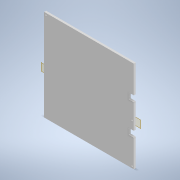
# Autodesk Inventor part: CoverPSU
Saved by Autodesk Inventor 2022 (Build 260153000, 153)
## iProperties
Created: 2022-01-15
Part Number: CoverPSU
Material: Generic
Document SubType Name: Modeling
Designer: siwat
Density: 1 g/cm^3
Appearance: Default
VLDS_Profile: Default Part
VLDS_TimeStamp: 2022-02-27
VLDS_FailCnt: 1
VLDS_AcceptCnt: 0
Author: siwat
Autodesk Inventor part; units mm, degrees
ref_plane "YZ Plane" through (0, 0, 0) normal (1, 0, 0) x (0, 1, 0)
ref_plane "XZ Plane" through (0, 0, 0) normal (0, 1, 0) x (-1, 0, 0)
ref_plane "XY Plane" through (0, 0, 0) normal (0, 0, 1) x (1, 0, 0)
ref_plane "Work Plane1" through (0, 0, 0) normal (0, 0, 1) x (1, 0, 0)
sketch "Sketch1" plane through (0, 0, 0) normal (0, 0, 1) x (1, 0, 0)
  line L0 (67.3785, -57.1866) -> (-67.4215, -57.1866)
  line L1 (-67.4215, -57.1866) -> (-67.4215, 80.2134)
  line L2 (-67.4215, 80.2134) -> (67.3785, 80.2134)
  line L3 (67.3785, 80.2134) -> (67.3785, -57.1866)
  circle A0 centre (64.6972, 5.0885) radius 1
  circle A1 centre (-64.8231, 77.3114) radius 1
  circle A2 centre (64.7712, -54.4524) radius 1
  point P0 (0, 0)
  dimension "d0" = 2
  dimension "d1" = 2
  dimension "d4" = 2
  dimension "d11" = 137.4
  dimension "d12" = 134.8
  constraints: 8 end point, 3 centre point, 2 parallel, 1 horizontal, 1 perpendicular
  measures "d0" diameter of A0
  measures "d1" diameter of A1
  measures "d4" diameter of A2
  measures "d11" distance of L2.end L0.start
  measures "d12" distance of L1.end L2.end
extrude "Extrusion1" add sketch "Sketch1" along normal blind 3
sketch "Sketch2" plane through (0, 0, 3) normal (0, 0, 1) x (1, 0, 0)
  line L0 (67.3785, -57.1866) -> (67.3785, 80.2134) projected
  line L1 (67.3785, -16.1531) -> (59.3785, -16.1531)
  line L2 (59.3785, -16.1531) -> (59.3785, -7.1531)
  line L3 (59.3785, -7.1531) -> (67.3785, -7.1531)
  line L4 (67.3785, -7.1531) -> (67.3785, -16.1531)
  line L5 (67.3785, 29.9305) -> (59.3785, 29.9305)
  line L6 (59.3785, 29.9305) -> (59.3785, 38.9305)
  line L7 (59.3785, 38.9305) -> (67.3785, 38.9305)
  line L8 (67.3785, 38.9305) -> (67.3785, 29.9305)
  point P0 (0, 0)
  dimension "d5" = 8
  dimension "d6" = 9
  dimension "d7" = 8
  dimension "d8" = 9
  constraints: 16 end point, 4 parallel, 2 horizontal, 2 perpendicular, 2 point on line
  measures "d5" distance of L2.end L3.end
  measures "d6" distance of L1.end L2.end
  measures "d7" distance of L6.end L7.end
  measures "d8" distance of L5.end L6.end
extrude "Extrusion2" cut sketch "Sketch2" against normal through all
body "Solid1"
